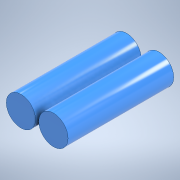
# Autodesk Inventor part: battery_2s
Saved by Autodesk Inventor 2021 (Build 250183000, 183)
## iProperties
Created: 2020-12-16
Part Number: battery_2s
Material: Generic
Document SubType Name: Modeling
Designer: oskar
Density: 1 g/cm^3
Appearance: Default
Author: oskar
Autodesk Inventor part; units mm, degrees
ref_plane "YZ Plane" through (0, 0, 0) normal (1, 0, 0) x (0, 1, 0)
ref_plane "XZ Plane" through (0, 0, 0) normal (0, 1, 0) x (-1, 0, 0)
ref_plane "XY Plane" through (0, 0, 0) normal (0, 0, 1) x (1, 0, 0)
sketch "Sketch1" plane through (0, 0, 0) normal (0, 0, 1) x (1, 0, 0)
  circle A0 centre (-20, 0) radius 9
  circle A1 centre (0, 0) radius 9
  line L0 (-36.6, 0) -> (16.6, 0) construction
  dimension "d0" = 18
  dimension "d1" = 18
  dimension "d2" = 20
  constraints: 2 centre point, 1 point on line
  measures "d0" diameter of A1
  measures "d1" diameter of A0
  measures "d2" distance of A1.centre A0.centre
extrude "Extrusion1" add sketch "Sketch1" along normal blind 65
equation "\"d1\" = d0"
body "Solid1"
